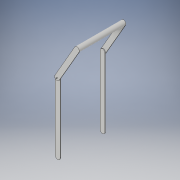
# Autodesk Inventor part: cart handle
Saved by Autodesk Inventor 2019 (Build 230136000, 136)
## iProperties
Created: 2018-12-09
Part Number: cart handle
Material: Generic
Document SubType Name: Modeling
Designer: Tiberus
Density: 1 g/cm^3
Appearance: Default
Author: Tiberus
Autodesk Inventor part; units mm, degrees
ref_plane "YZ Plane" through (0, 0, 0) normal (1, 0, 0) x (0, 1, 0)
ref_plane "XZ Plane" through (0, 0, 0) normal (0, 1, 0) x (-1, 0, 0)
ref_plane "XY Plane" through (0, 0, 0) normal (0, 0, 1) x (1, 0, 0)
sketch "Sketch1" plane through (0, 0, 0) normal (0, 0, 1) x (1, 0, 0)
  line L0 (25.4, 0) -> (25.4, 359.664)
  line L1 (0, 359.664) -> (0, 0)
  arc A0 (0, 0) -> (25.4, 0) centre (12.7, 0) ccw
  arc A1 (25.4, 359.664) -> (0, 359.664) centre (12.7, 359.664) ccw
  constraints: 4 end point, 4 point on circle, 4 tangent, 2 centre point, 1 parallel
sketch "Sketch2" plane through (0, 0, 0) normal (0, 0, 1) x (1, 0, 0)
  line L0 (-287.7794, 186.1816) -> (71.8846, 186.1816) construction
  arc A0 (25.4, 359.664) -> (0, 359.664) centre (12.7, 359.664) ccw projected
  arc A1 (18.9244, 348.5939) -> (19.1748, 348.7385) centre (12.7, 359.664) ccw
  arc A2 (6.4756, 370.7341) -> (6.2252, 370.5895) centre (12.7, 359.664) ccw
  line L1 (12.7, 359.664) -> (220.472, 359.664) construction
  line L2 (23.6985, 353.314) -> (127.5845, 533.2498)
  line L3 (105.5875, 545.9498) -> (1.7015, 366.014)
  arc A3 (1.7015, 366.014) -> (23.6985, 353.314) centre (12.7, 359.664) ccw
  arc A4 (127.5845, 533.2498) -> (105.5875, 545.9498) centre (116.586, 539.5998) ccw
  point P0 (0, 0)
  constraints: 10 point on circle, 8 end point, 4 centre point, 4 tangent, 2 horizontal, 1 coincident, 1 parallel, 1 point on line
extrude "Extrusion1" add sketch "Sketch2" along normal blind 3.175
extrude "Extrusion2" add sketch "Sketch1" against normal blind 3.175
sketch "Sketch3" plane through (0, 0, 3.175) normal (0, 0, 1) x (1, 0, 0)
  circle A0 centre (12.7, 359.664) radius 2.5797
  point P0 (0, 0)
  dimension "d12" = 5.1594
  constraints: 1 centre point
  measures "d12" diameter of A0
extrude "Extrusion3" add sketch "Sketch3" along normal blind 3.175
sketch "Sketch4" plane through (0, 0, 0) normal (0, 0, -1) x (-1, 0, 0)
  arc A0 (-105.5875, 545.9498) -> (-127.5845, 533.2498) centre (-116.586, 539.5998) ccw projected
  circle A1 centre (-116.586, 539.5998) radius 12.7
  point P0 (0, 0)
  constraints: 1 centre point, 1 coincident
extrude "Extrusion4" add sketch "Sketch4" along normal blind 120.65
ref_plane "Work Plane2" through (127.5845, 533.2498, -119.0625) normal (0, 0, 1) x (1, 0, 0)
ref_plane "Work Plane1" through (127.5845, 533.2498, 1.5875) normal (0, 0, 1) x (1, 0, 0)
mirror "Mirror1" about plane through (127.5845, 533.2498, -119.0625) normal (0, 0, 1) of "Extrusion4", "Extrusion1", "Extrusion2"
body "Solid1"
